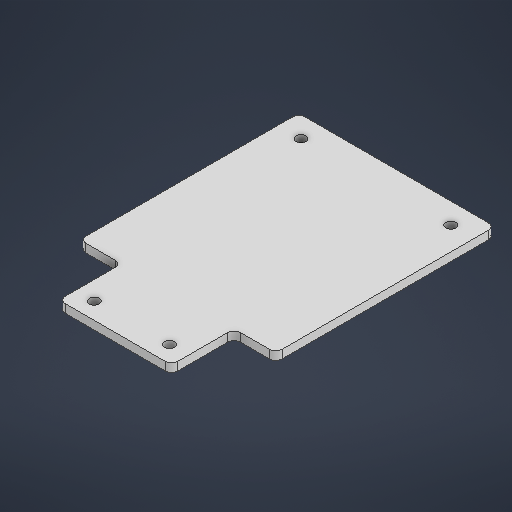
# Autodesk Inventor part: 1.5_base_2
Saved by Autodesk Inventor 2025 (Build 290162010, 162A)
## iProperties
Created: 2024-05-22
Part Number: 1.5_base_2
Material: Generic
Document SubType Name: Modeling
Designer: Garfieldcmix
Density: 1 g/cm^3
Appearance: Default
Author: Garfieldcmix
Autodesk Inventor part; units mm, degrees
ref_plane "YZ Plane" through (0, 0, 0) normal (1, 0, 0) x (0, 1, 0)
ref_plane "XZ Plane" through (0, 0, 0) normal (0, 1, 0) x (-1, 0, 0)
ref_plane "XY Plane" through (0, 0, 0) normal (0, 0, 1) x (1, 0, 0)
derived "Car_Plan.ipt"
sketch "Car_Sketch" plane through (0, 0, 0) normal (0, 1, 0) x (-1, 0, 0)
  line L0 (0, 0) -> (94, 0)
  line L1 (0, 0) -> (0, 105)
  line L2 (94, 0) -> (94, 105)
  line L3 (0, 105) -> (20, 105)
  line L4 (20, 105) -> (20, 190)
  line L5 (20, 190) -> (74, 190)
  line L6 (74, 190) -> (74, 105)
  line L7 (74, 105) -> (94, 105)
  line L8 (-5, 68) -> (-5, 0)
  line L9 (-5, 0) -> (-32, 0)
  line L10 (-32, 0) -> (-32, 68)
  line L11 (-32, 68) -> (-5, 68)
  line L12 (47, 190) -> (47, 0) construction
  line L13 (126, 68) -> (99, 68)
  line L14 (99, 68) -> (99, 0)
  line L15 (126, 0) -> (126, 68)
  line L16 (99, 0) -> (126, 0)
  line L17 (-5, 34) -> (99, 34) construction
  line L18 (0, 95) -> (94, 95) construction
  line L19 (-5, 190) -> (-32, 190)
  line L20 (-32, 122) -> (-5, 122)
  line L21 (-32, 190) -> (-32, 122)
  line L22 (-5, 122) -> (-5, 190)
  line L23 (-5, 156) -> (99, 156) construction
  line L24 (126, 122) -> (99, 122)
  line L25 (126, 190) -> (126, 122)
  line L26 (99, 190) -> (126, 190)
  line L27 (99, 122) -> (99, 190)
  line L28 (0, 156) -> (47, 34) construction
  line L29 (94, 156) -> (47, 34) construction
  line L30 (0, 156) -> (-174.2341, 34) construction
  line L31 (-5, 34) -> (-174.2341, 34) construction
  line L32 (8.9873, 132.6713) -> (47, 141.55) construction
  line L33 (85.0127, 132.6713) -> (47, 141.55) construction
sketch "Base" plane through (0, 0, 0) normal (0, 1, 0) x (-1, 0, 0)
  line L0 (0, 0) -> (0, 105) projected
  line L1 (0, 105) -> (20, 105) projected
  line L2 (20, 105) -> (20, 190) projected
  line L3 (74, 190) -> (74, 105) projected
  line L4 (74, 105) -> (94, 105) projected
  line L5 (94, 0) -> (94, 105) projected
  line L6 (0, 0) -> (94, 0) projected
  line L7 (74, 135) -> (20, 135)
  circle A0 centre (29, 127) radius 2.4
  circle A1 centre (65, 127) radius 2.4
  circle A2 centre (11.1, 10) radius 2.4
  circle A3 centre (82.9, 10) radius 2.4
  dimension "d76" = 30
  dimension "d77" = 4.8
  dimension "d78" = 4.8
  dimension "d79" = 9
  dimension "d80" = 22
  dimension "d81" = 22
  dimension "d82" = 9
  dimension "d83" = 4.8
  dimension "d84" = 4.8
  dimension "d85" = 10
  dimension "d86" = 11.1
  dimension "d87" = 10
  dimension "d88" = 11.1
  constraints: 4 centre point, 2 end point, 2 point on line, 1 perpendicular
  measures "d76" distance between parallel lines of L1 L7
  measures "d77" diameter of A0
  measures "d78" diameter of A1
  measures "d79" distance from line of L2 A0.centre
  measures "d80" distance from line of L1 A0.centre
  measures "d81" distance from line of A1.centre L4
  measures "d82" distance from line of L3 A1.centre
  measures "d83" diameter of A2
  measures "d84" diameter of A3
  measures "d85" distance from line of L6 A2.centre
  measures "d86" distance from line of L0 A2.centre
  measures "d87" distance from line of L6 A3.centre
  measures "d88" distance from line of L5 A3.centre
extrude "Extrusion1" add sketch "Base" along normal blind 4
fillet "Fillet2" radius 3 8 edges at (-20, 2, 105) (0, 2, 105) (0, 2, 0) (-94, 2, 0) (-94, 2, 105) (-74, 2, 105) (-74, 2, 135) (-20, 2, 135)
body "Solid1"
